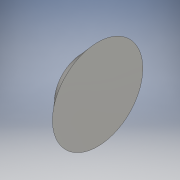
# Autodesk Inventor part: Handle Gearbox
Saved by Autodesk Inventor 2016 (Build 200138000, 138)
## iProperties
Created: 2017-08-08
Part Number: Handle Gearbox
Material: PC/ABS Plastic
Document SubType Name: Modeling
Designer: M227562
Density: 0.357273 g/cm^3
Appearance: Smooth - White
Author: M227562
Autodesk Inventor part; units mm, degrees
ref_plane "YZ Plane" through (0, 0, 0) normal (1, 0, 0) x (0, 1, 0)
ref_plane "XZ Plane" through (0, 0, 0) normal (0, 1, 0) x (-1, 0, 0)
ref_plane "XY Plane" through (0, 0, 0) normal (0, 0, 1) x (1, 0, 0)
sketch "Sketch2" plane through (0, 0, 0) normal (0, 1, 0) x (-1, 0, 0)
  line L0 (0, 0) -> (0, -65)
  line L1 (0, 0) -> (22, 0)
  line L2 (22, 0) -> (22, -40.3)
  line L3 (22, -40.3) -> (0, -65)
  dimension "d4" = 65
  dimension "d5" = 22
  dimension "d6" = 40.3
  constraints: 8 end point, 1 horizontal, 1 perpendicular, 1 vertical
  measures "d4" distance of L0.start L0.end
  measures "d5" distance of L0.start L1.end
  measures "d6" distance of L1.end L2.end
revolve "Revolution1" add sketch "Sketch2" angle 360 about axis through (0, 0, 0) along (-1, 0, 0)
sketch "Sketch3" plane through (-22, 0, 0) normal (-1, 0, 0) x (0, 0, 1)
  circle A0 centre (0, 0) radius 40.3 projected
  line L0 (0, 40.3) -> (0, 64.3)
  line L1 (0, 64.3) -> (-7.5, 64.3)
  line L2 (-7.5, 64.3) -> (-7.5, 39.596)
  line L3 (0, 64.3) -> (7.4, 64.3)
  line L4 (7.4, 64.3) -> (7.5, 39.596)
  arc A1 (7.5, 39.596) -> (-7.5, 39.596) centre (0, 0) ccw
  dimension "d11" = 24
  dimension "d12" = 7.5
  dimension "d13" = 7.4
  constraints: 10 end point, 6 point on circle, 2 perpendicular, 1 centre point, 1 point on line, 1 vertical
  measures "d11" distance of L0.start L0.end
  measures "d12" distance of L0.end L1.end
  measures "d13" distance of L0.end L3.end
extrude "Extrusion1" cut sketch "Sketch3" against normal blind 10 contours A0 L0 L3 L4 | L2 L1 L0 A0
body "Solid1"
